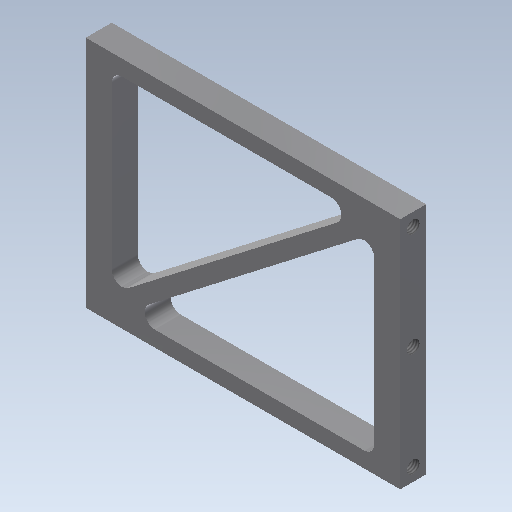
# Autodesk Inventor part: Link_front_diagonal
Saved by Autodesk Inventor 2020.4 (Build 244396000, 396)
## iProperties
Created: 2016-06-03
Part Number: Link_front_diagonal
Material: アルミニウム 2014-T4
Document SubType Name: Modeling
Designer: hiroaki
Density: 2.8 g/cm^3
Appearance: 滑らか - 淡い灰色
Mass: 12.996 g
Surface Area: 43.7686 cm^2
Volume: 4.64142 cm^3
Description: A2017 T5
Author: hiroaki
Title: リンク_ふくらはぎ_サブフレーム_1_1
Autodesk Inventor part; units mm, degrees
ref_plane "YZ Plane" through (0, 0, 0) normal (1, 0, 0) x (0, 1, 0)
ref_plane "XZ Plane" through (0, 0, 0) normal (0, 1, 0) x (-1, 0, 0)
ref_plane "XY Plane" through (0, 0, 0) normal (0, 0, 1) x (1, 0, 0)
sketch "スケッチ1" plane through (0, 0, 0) normal (0, 0, 1) x (1, 0, 0)
  line L0 (-30.25, 22.5) -> (30.25, 22.5)
  line L1 (30.25, 22.5) -> (30.25, -22.5)
  line L2 (30.25, -22.5) -> (-30.25, -22.5)
  line L3 (-30.25, -22.5) -> (-30.25, 22.5)
  line L4 (-25.25, 19.5) -> (25.25, 19.5) construction
  line L5 (25.25, 19.5) -> (25.25, -19.5) construction
  line L6 (25.25, -19.5) -> (-25.25, -19.5) construction
  line L7 (-25.25, -19.5) -> (-25.25, 19.5) construction
  line L8 (25.25, 19.5) -> (-25.25, -19.5) construction
  line L9 (-25.25, -17.6048) -> (-25.25, 19.5)
  line L10 (-25.25, 19.5) -> (22.7959, 19.5)
  line L11 (22.7959, 19.5) -> (-25.25, -17.6048)
  line L12 (-22.7959, -19.5) -> (25.25, -19.5)
  line L13 (25.25, -19.5) -> (25.25, 17.6048)
  line L14 (25.25, 17.6048) -> (-22.7959, -19.5)
  line L15 (-30.25, 20) -> (30.25, 20) construction
  line L16 (30.25, -20) -> (-30.25, -20) construction
  line L17 (30.25, 20) -> (30.25, -20) construction
  point P0 (0, 0)
  point P1 (0, 19.5)
  point P2 (0, 22.5)
  point P3 (25.25, 0)
  point P4 (30.25, 0)
  dimension "d0" = 5
  dimension "d1" = 3
  dimension "d2" = 1.5
  dimension "d3" = 40
  dimension "d4" = 2.5
  dimension "d19" = 60.5
  constraints: 36 end point, 6 parallel, 5 collinear, 5 horizontal, 5 midpoint, 4 perpendicular, 4 point on line, 2 horizontal alignment, 2 vertical alignment, 1 vertical, 1 other
  measures "d0" distance between parallel lines of L3 L7
  measures "d1" distance between parallel lines of L0 L4
  measures "d2" distance between parallel lines of L8 L11
  measures "d3" distance between parallel lines of L16 L15
  measures "d4" distance between parallel lines of L2 L16
  measures "d19" distance of L0.start L0.end
extrude "押し出し1" add sketch "スケッチ1" along normal blind 5
sketch "スケッチ2" plane through (30.25, -22.5, 0) normal (1, 0, 0) x (0, 0, -1)
  line L0 (0, 45) -> (-5, 45) projected
  line L1 (-5, 0) -> (-5, 45) projected
  line L2 (0, 22.5) -> (-5, 22.5) construction
  point P0 (-2.5, 2.5)
  point P1 (-2.5, 22.5)
  point P2 (-2.5, 42.5)
  point P3 (-2.5, 45)
  dimension "d7" = 40
  constraints: 3 midpoint, 3 vertical alignment, 2 end point, 1 symmetric about line
  measures "d7" distance of point (-2.5, 42.5) point (-2.5, 2.5)
hole "穴1" at (30.25, -20, 2.5) at (30.25, 0, 2.5) at (30.25, 20, 2.5) direction (-1, 0, 0) diameter 2.459 depth 3 thread size "M3x0.5" class "6H" standard "ISO Metric profile"
mirror "ミラー1" about plane through (0, 0, 0) normal (1, 0, 0) of "穴1"
fillet "フィレット1" radius 2 6 edges at (-22.7959, -19.5, 2.5) (-25.25, -17.6048, 2.5) (25.25, 17.6048, 2.5) (25.25, -19.5, 2.5) (-25.25, 19.5, 2.5) (22.7959, 19.5, 2.5)
equation "\"d3\" = d11_1"
equation "\"d7\" = d3"
equation "\"d11_1\" = 40"
